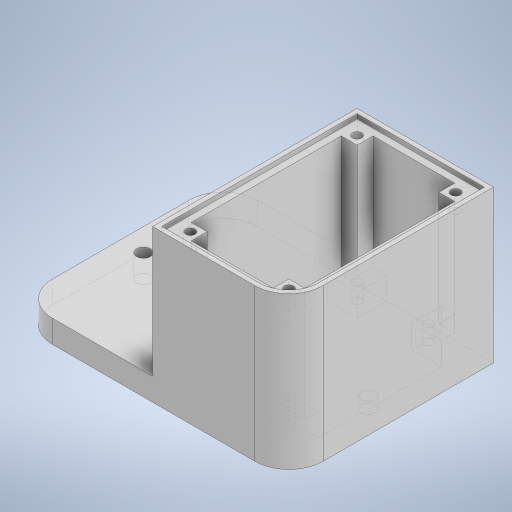
# Autodesk Inventor part: Gehäuse
Saved by Autodesk Inventor 2024.2 (Build 282272000, 272)
## iProperties
Created: 2023-10-24
Part Number: Gehäuse
Material: Generisch
Document SubType Name: Modeling
Designer: Pieber
Density: 1 g/cm^3
Appearance: Vorgabe
Author: Pieber
Autodesk Inventor part; units mm, degrees
ref_plane "YZ Plane" through (0, 0, 0) normal (1, 0, 0) x (0, 1, 0)
ref_plane "XZ Plane" through (0, 0, 0) normal (0, 1, 0) x (-1, 0, 0)
ref_plane "XY Plane" through (0, 0, 0) normal (0, 0, 1) x (1, 0, 0)
sketch "Skizze61" plane through (0, 0, 0) normal (0, 0, 1) x (1, 0, 0)
  line L0 (30, -45) -> (-30, -45)
  line L1 (-30, -45) -> (-30, 45)
  line L2 (-30, 45) -> (30, 45)
  line L3 (30, 45) -> (30, -45)
  line L4 (30, -45) -> (-30, 45) construction
  line L5 (-30, -45) -> (30, 45) construction
  point P0 (0, 0)
  dimension "d159" = 60
  dimension "d160" = 90
  constraints: 12 end point, 2 midpoint, 2 parallel, 1 horizontal, 1 perpendicular
  measures "d159" distance of L1.end L2.end
  measures "d160" distance of L0.end L1.end
extrude "Extrusion54" add sketch "Skizze61" along normal blind 65
shell "Wandung3" thickness 5 removed faces 1 at (-10, 15, 65)
sketch "Sketch69" plane through (-30, -45, 0) normal (-1, 0, 0) x (0, 0, 1)
  line L0 (0, 90) -> (65, 90) projected
  line L1 (0, 0) -> (65, 0) projected
  line L2 (0, 90) -> (10, 90)
  line L3 (10, 90) -> (10, 0)
  line L4 (10, 0) -> (0, 0)
  line L5 (0, 0) -> (0, 90)
  point P0 (0, 45)
  dimension "d192" = 10
  constraints: 8 end point, 2 parallel, 1 horizontal, 1 perpendicular, 1 point on line
  measures "d192" distance of L3.end L4.end
extrude "Extrusion61" add sketch "Sketch69" along normal blind 59
sketch "Sketch71" plane through (0, 0, 0) normal (0, 0, -1) x (-1, 0, 0)
  line L0 (-8, -33.57) -> (-12, -33.57)
  line L1 (-12, -33.57) -> (-12, -26.57)
  line L2 (-12, -26.57) -> (-8, -26.57)
  line L3 (-8, -26.57) -> (-8, -33.57)
  line L4 (89, 45) -> (89, -45) projected
  line L5 (-30, -45) -> (89, -45) projected
  point P0 (0, 0)
  dimension "d199" = 4
  dimension "d200" = 7
  dimension "d201" = 97
  dimension "d202" = 11.43
  constraints: 8 end point, 2 parallel, 1 horizontal, 1 perpendicular
  measures "d199" distance of L1.end L2.end
  measures "d200" distance of L0.end L1.end
  measures "d201" distance between parallel lines of L4 L3
  measures "d202" distance between parallel lines of L5 L0
extrude "Extrusion63" cut sketch "Sketch71" against normal blind 10
sketch "Sketch70" plane through (0, 0, 0) normal (0, 0, -1) x (-1, 0, 0)
  line L0 (30, 45) -> (89, 45) projected
  line L1 (30, -45) -> (89, -45) projected
  line L2 (89, 45) -> (69, 45)
  line L3 (69, 45) -> (69, -45)
  line L4 (69, -45) -> (89, -45)
  line L5 (89, -45) -> (89, 45)
  circle A0 centre (79, 0) radius 3
  point P0 (0, 0)
  dimension "d195" = 20
  dimension "d196" = 6
  constraints: 8 end point, 2 parallel, 1 centre point, 1 horizontal, 1 perpendicular, 1 point on line
  measures "d195" distance of L4.end L3.end
  measures "d196" diameter of A0
extrude "Extrusion62" cut sketch "Sketch70" against normal through all contours A0
sketch "Sketch72" plane through (0, 0, 0) normal (0, 0, -1) x (-1, 0, 0)
  circle A0 centre (-20, 0) radius 3
  line L0 (-30, -45) -> (-30, 45) projected
  point P0 (0, 0)
  dimension "d205" = 6
  dimension "d206" = 10
  constraints: 1 centre point
  measures "d205" diameter of A0
  measures "d206" distance from line of L0 A0.centre
extrude "Extrusion64" cut sketch "Sketch72" against normal through all
sketch "Sketch73" plane through (0, 0, 0) normal (0, 0, -1) x (-1, 0, 0)
  point P0 (0, 0)
fillet "Rundung1" radius 15 2 edges at (-89, 45, 5) (-89, -45, 5)
fillet "Rundung2" radius 15 1 edges at (30, -45, 32.5)
sketch "Skizze78" plane through (-25, 40, 5) normal (0, 0, 1) x (1, 0, 0)
  line L0 (0, 0) -> (7, 0)
  line L1 (7, 0) -> (7, -7)
  line L2 (7, -7) -> (0, -7)
  line L3 (0, -7) -> (0, 0)
  line L4 (50, -80) -> (50, 0) projected
  line L5 (50, 0) -> (43, 0)
  line L6 (43, 0) -> (43, -7)
  line L7 (43, -7) -> (50, -7)
  line L8 (50, -7) -> (50, 0)
  line L9 (50, -80) -> (0, -80) projected
  line L10 (0, -80) -> (7, -80)
  line L11 (7, -80) -> (7, -73)
  line L12 (7, -73) -> (0, -73)
  line L13 (0, -73) -> (0, -80)
  line L14 (50, -80) -> (43, -80)
  line L15 (43, -80) -> (43, -73)
  line L16 (43, -73) -> (50, -73)
  line L17 (50, -73) -> (50, -80)
  point P0 (25, -40)
  dimension "d239" = 7
  dimension "d240" = 7
  dimension "d241" = 7
  dimension "d242" = 7
  dimension "d243" = 7
  dimension "d244" = 7
  dimension "d245" = 7
  dimension "d246" = 7
  constraints: 32 end point, 8 parallel, 4 horizontal, 4 perpendicular
  measures "d239" distance of L1.end L2.end
  measures "d240" distance of L0.end L1.end
  measures "d241" distance of L7.end L6.end
  measures "d242" distance of L6.end L5.end
  measures "d243" distance of L12.end L11.end
  measures "d244" distance of L11.end L10.end
  measures "d245" distance of L15.end L16.end
  measures "d246" distance of L14.end L15.end
extrude "Extrusion68" add sketch "Skizze78" along normal up to surface (60 mm away)
sketch "Skizze79" plane through (0, 0, 65) normal (0, 0, 1) x (1, 0, 0)
  line L0 (30, 45) -> (-30, 45) projected
  line L1 (-30, -45) -> (15, -45) projected
  line L2 (-30, 45) -> (-28, 45)
  line L3 (-28, 45) -> (-28, -45)
  line L4 (-28, -45) -> (-30, -45)
  line L5 (-30, -45) -> (-30, 45)
  line L6 (30, -30) -> (30, 45) projected
  line L7 (-28, 45) -> (30, 45)
  line L8 (30, 45) -> (30, 43)
  line L9 (30, 43) -> (-28, 43)
  line L10 (-28, 43) -> (-28, 45)
  line L11 (30, 43) -> (28, 43)
  line L12 (28, 43) -> (28, -30)
  line L13 (28, -30) -> (30, -30)
  line L14 (30, -30) -> (30, 43)
  line L15 (-28, -45) -> (15, -45)
  line L16 (15, -45) -> (15, -43)
  line L17 (15, -43) -> (-28, -43)
  line L18 (-28, -43) -> (-28, -45)
  arc A0 (15, -45) -> (30, -30) centre (15, -30) ccw projected
  arc A1 (15, -45) -> (30, -30) centre (15, -30) ccw
  arc A2 (15, -43) -> (28, -30) centre (15, -30) ccw
  point P0 (0, 0)
  point P1 (-28, -43)
  point P2 (29, -30)
  dimension "d249" = 2
  dimension "d250" = 2
  dimension "d251" = 2
  dimension "d252" = 2
  dimension "d268" = 75
  constraints: 32 end point, 8 parallel, 4 horizontal, 4 perpendicular, 4 point on circle, 2 centre point, 2 coincident, 2 point on line, 1 midpoint
  measures "d249" distance of L3.end L4.end
  measures "d250" distance of L7.end L8.end
  measures "d251" distance of L13.end L12.end
  measures "d252" distance of L16.end L15.end
  measures "d268" distance from line of L0 point (29, -30)
extrude "Extrusion69" add sketch "Skizze79" along normal blind 2 contours L6 L9 L3 L0 | L3 L1 L5 L0 | L6 L13 L12 L9 | A0 L16 A2 L13 | L17 L16 L1 L3
sketch "Skizze80" plane through (-18, -40, 5) normal (0, 0, 1) x (1, 0, 0)
  line L0 (0, 80) -> (36, 80) projected
  line L1 (0, 80) -> (6, 80)
  line L2 (6, 80) -> (6, 67)
  line L3 (6, 67) -> (0, 67)
  line L4 (0, 67) -> (0, 80)
  line L5 (-7, 7) -> (-7, 73) projected
  line L6 (0, 67) -> (-7, 67)
  line L7 (-7, 67) -> (-7, 73)
  line L8 (-7, 73) -> (0, 73)
  line L9 (0, 73) -> (0, 67)
  line L10 (36, 73) -> (36, 80) projected
  line L11 (36, 80) -> (30, 80)
  line L12 (30, 80) -> (30, 67)
  line L13 (30, 67) -> (36, 67)
  line L14 (36, 67) -> (36, 80)
  line L15 (43, 7) -> (43, 73) projected
  line L16 (36, 67) -> (43, 67)
  line L17 (43, 67) -> (43, 73)
  line L18 (43, 73) -> (36, 73)
  line L19 (36, 73) -> (36, 67)
  line L20 (-7, 7) -> (6, 7)
  line L21 (6, 7) -> (6, 13)
  line L22 (6, 13) -> (-7, 13)
  line L23 (-7, 13) -> (-7, 7)
  line L24 (36, 0) -> (0, 0) projected
  line L25 (6, 7) -> (0, 7)
  line L26 (0, 7) -> (0, 0)
  line L27 (0, 0) -> (6, 0)
  line L28 (6, 0) -> (6, 7)
  line L29 (43, 7) -> (30, 7)
  line L30 (30, 7) -> (30, 13)
  line L31 (30, 13) -> (43, 13)
  line L32 (43, 13) -> (43, 7)
  line L33 (36, 0) -> (30, 0)
  line L34 (30, 0) -> (30, 7)
  line L35 (30, 7) -> (36, 7)
  line L36 (36, 7) -> (36, 0)
  point P0 (18, 40)
  point P1 (43, 7)
  point P2 (43, 13)
  point P3 (30, 0)
  point P4 (-7, 13)
  point P5 (6, 0)
  point P6 (36, 73)
  point P7 (0, 73)
  point P8 (-7, 67)
  dimension "d255" = 6
  dimension "d256" = 13
  dimension "d257" = 6
  dimension "d258" = 13
  dimension "d259" = 7
  dimension "d260" = 6
  dimension "d261" = 13
  dimension "d262" = 6
  dimension "d263" = 6
  dimension "d264" = 13
  dimension "d265" = 6
  dimension "d274" = 13
  constraints: 64 end point, 16 parallel, 8 horizontal, 8 perpendicular, 3 point on line
  measures "d255" distance of L2.end L3.end
  measures "d256" distance of L1.end L2.end
  measures "d257" distance of L13.end L12.end
  measures "d258" distance of L12.end L11.end
  measures "d259" distance of L18.end L15.end
  measures "d260" distance of L15.end L16.end
  measures "d261" distance of L22.end L21.end
  measures "d262" distance of L21.end L20.end
  measures "d263" distance of L27.end L24.end
  measures "d264" distance of L30.end L31.end
  measures "d265" distance of L29.end L30.end
  measures "d274" distance between parallel lines of L24 L22
extrude "Extrusion70" add sketch "Skizze80" along normal blind 10 contours L0 L2 L3 L4 | L4 L6 L5 L8 | L0 L10 L14 L13 L12 | L18 L15 L16 L14 | L22 L21 L20 L5 | L15 L29 L30 L31 | L20 L28 L24 L26 | L36 L24 L34 L29
sketch "Skizze81" plane through (0, 0, 65) normal (0, 0, 1) x (1, 0, 0)
  circle A0 centre (-21.7, -36.7) radius 2
  line L0 (-18, -33) -> (-18, -40) projected
  line L1 (-25, -33) -> (-18, -33) projected
  point P0 (0, 0)
  dimension "d269" = 3.7
  dimension "d270" = 3.7
  dimension "d271" = 4
  constraints: 1 centre point
  measures "d269" distance from line of L0 A0.centre
  measures "d270" distance from line of L1 A0.centre
  measures "d271" diameter of A0
extrude "Extrusion71" cut sketch "Skizze81" against normal blind 7
mirror "Spiegeln11" about plane through (0, 0, 0) normal (1, 0, 0) of "Extrusion71"
mirror "Spiegeln12" about plane through (0, 0, 0) normal (0, 1, 0) of "Extrusion71", "Spiegeln11"
sketch "Skizze82" plane through (-18, -40, 15) normal (0, 0, 1) x (1, 0, 0)
  circle A0 centre (33.7, 9.3) radius 2
  line L0 (30, 13) -> (30, 0) projected
  line L1 (43, 13) -> (30, 13) projected
  point P0 (18, 40)
  dimension "d275" = 4
  dimension "d276" = 3.7
  dimension "d277" = 3.7
  constraints: 1 centre point
  measures "d275" diameter of A0
  measures "d276" distance from line of L0 A0.centre
  measures "d277" distance from line of L1 A0.centre
extrude "Extrusion72" cut sketch "Skizze82" against normal blind 7
mirror "Spiegeln13" about plane through (0, 0, 0) normal (0, 1, 0) of "Extrusion72"
mirror "Spiegeln14" about plane through (0, 0, 0) normal (1, 0, 0) of "Extrusion72", "Spiegeln13"
